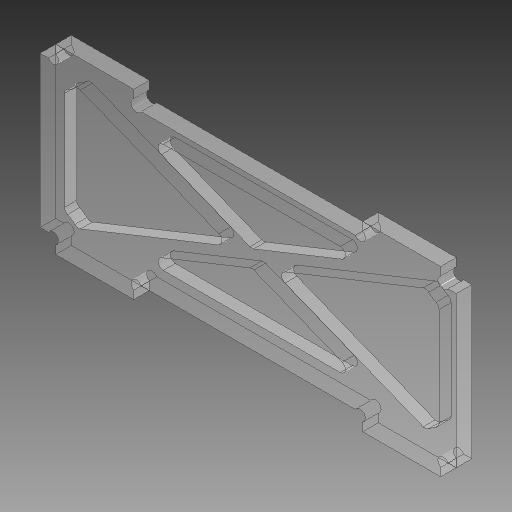
# Autodesk Inventor part: 平行サス板4
Saved by Autodesk Inventor 2020 (Build 240168000, 168)
## iProperties
Created: 2019-09-03
Part Number: 平行サス板4
Material: ポリカーボネート、クリア
Document SubType Name: Modeling
Designer: 雪村
Density: 1.2 g/cm^3
Appearance: ポリカーボネート - クリア
Mass: 5.70734 g
Surface Area: 64.8254 cm^2
Volume: 4.75612 cm^3
Description: ポリカ 3t
Author: 雪村
Autodesk Inventor part; units mm, degrees
ref_plane "YZ Plane" through (0, 0, 0) normal (1, 0, 0) x (0, 1, 0)
ref_plane "XZ Plane" through (0, 0, 0) normal (0, 1, 0) x (-1, 0, 0)
ref_plane "XY Plane" through (0, 0, 0) normal (0, 0, 1) x (1, 0, 0)
sketch "スケッチ1" plane through (0, 0, 0) normal (0, 0, 1) x (1, 0, 0)
  line L0 (0, 0) -> (80, 0)
  line L1 (80, 0) -> (80, 29)
  line L2 (80, 29) -> (0, 29)
  line L3 (0, 29) -> (0, 0)
  line L4 (3, 29) -> (18, 29)
  line L5 (18, 29) -> (18, 32)
  line L6 (18, 32) -> (3, 32)
  line L7 (3, 32) -> (3, 29)
  line L8 (77, 29) -> (62, 29)
  line L9 (62, 29) -> (62, 32)
  line L10 (62, 32) -> (77, 32)
  line L11 (77, 32) -> (77, 29)
  line L12 (3, 0) -> (18, 0)
  line L13 (18, 0) -> (18, -3)
  line L14 (18, -3) -> (3, -3)
  line L15 (3, -3) -> (3, 0)
  line L16 (62, 0) -> (77, 0)
  line L17 (77, 0) -> (77, -3)
  line L18 (77, -3) -> (62, -3)
  line L19 (62, -3) -> (62, 0)
  dimension "d0" = 29
  dimension "d1" = 80
  dimension "d2" = 15
  dimension "d3" = 3
  dimension "d4" = 15
  dimension "d5" = 3
  dimension "d6" = 15
  dimension "d7" = 3
  dimension "d8" = 15
  dimension "d9" = 3
  dimension "d10" = 3
  dimension "d11" = 3
  dimension "d12" = 3
  dimension "d13" = 3
  constraints: 40 end point, 10 horizontal, 10 vertical, 4 point on line
  measures "d0" distance of L1.end L0.end
  measures "d1" distance of L1.end L2.end
  measures "d2" distance of L6.end L5.end
  measures "d3" distance of L5.end L4.end
  measures "d4" distance of L9.end L10.end
  measures "d5" distance of L8.end L9.end
  measures "d6" distance of L13.end L14.end
  measures "d7" distance of L12.end L13.end
  measures "d8" distance of L17.end L18.end
  measures "d9" distance of L16.end L17.end
  measures "d10" distance between parallel lines of L1 L17
  measures "d11" distance between parallel lines of L15 L3
  measures "d12" distance between parallel lines of L3 L7
  measures "d13" distance between parallel lines of L1 L11
extrude "押し出し1" add sketch "スケッチ1" along normal blind 3
sketch "スケッチ2" plane through (0, 0, 3) normal (0, 0, 1) x (1, 0, 0)
  line L0 (3, 29) -> (0, 29) projected
  line L1 (3, 32) -> (3, 29) projected
  line L2 (18, 29) -> (18, 32) projected
  line L3 (62, 29) -> (18, 29) projected
  line L4 (62, 32) -> (62, 29) projected
  line L5 (77, 29) -> (77, 32) projected
  line L6 (80, 29) -> (77, 29) projected
  line L7 (77, 0) -> (80, 0) projected
  line L8 (77, -3) -> (77, 0) projected
  line L9 (62, 0) -> (62, -3) projected
  line L10 (18, 0) -> (62, 0) projected
  line L11 (18, -3) -> (18, 0) projected
  line L12 (0, 0) -> (3, 0) projected
  circle A0 centre (2.5, 29.5) radius 1.05
  circle A1 centre (18.5, 29.5) radius 1.05
  circle A2 centre (61.5, 29.5) radius 1.05
  circle A3 centre (77.5, 29.5) radius 1.05
  circle A4 centre (2.5, -0.5) radius 1.05
  circle A5 centre (18.5, -0.5) radius 1.05
  circle A6 centre (61.5, -0.5) radius 1.05
  circle A7 centre (77.5, -0.5) radius 1.05
  line L13 (3, 0) -> (3, -3) projected
  dimension "d16" = 2.1
  dimension "d17" = 2.1
  dimension "d18" = 2.1
  dimension "d19" = 2.1
  dimension "d20" = 2.1
  dimension "d21" = 2.1
  dimension "d22" = 2.1
  dimension "d23" = 2.1
  dimension "d24" = 0.5
  dimension "d25" = 0.5
  dimension "d26" = 0.5
  dimension "d27" = 0.5
  dimension "d28" = 0.5
  dimension "d29" = 0.5
  dimension "d30" = 0.5
  dimension "d31" = 0.5
  dimension "d32" = 0.5
  dimension "d33" = 0.5
  dimension "d34" = 0.5
  dimension "d35" = 0.5
  dimension "d36" = 0.5
  dimension "d37" = 0.5
  dimension "d38" = 0.5
  dimension "d39" = 0.5
  constraints: 8 centre point
  measures "d16" diameter of A0
  measures "d17" diameter of A1
  measures "d18" diameter of A2
  measures "d19" diameter of A3
  measures "d20" diameter of A4
  measures "d21" diameter of A5
  measures "d22" diameter of A6
  measures "d23" diameter of A7
  measures "d24" distance from line of L0 A0.centre
  measures "d25" distance from line of L1 A0.centre
  measures "d26" distance from line of L3 A1.centre
  measures "d27" distance from line of L2 A1.centre
  measures "d28" distance from line of L3 A2.centre
  measures "d29" distance from line of L4 A2.centre
  measures "d30" distance from line of L6 A3.centre
  measures "d31" distance from line of L5 A3.centre
  measures "d32" distance from line of A4.centre L12
  measures "d33" distance from line of L13 A4.centre
  measures "d34" distance from line of L10 A5.centre
  measures "d35" distance from line of L11 A5.centre
  measures "d36" distance from line of L10 A6.centre
  measures "d37" distance from line of L9 A6.centre
  measures "d38" distance from line of A7.centre L7
  measures "d39" distance from line of L8 A7.centre
extrude "押し出し2" cut sketch "スケッチ2" against normal through all
shell "シェル1" thickness 4 removed faces 2 at (33.1411, 9.6667, 3) at (46.8589, 19.3333, 0)
sketch "スケッチ3" plane through (0, 0, 3) normal (0, 0, 1) x (1, 0, 0)
  line L0 (76, 24.6779) -> (76, 4.3221) projected
  arc A0 (76, 4.3221) -> (72.6779, 1) centre (77.5, -0.5) ccw projected
  line L1 (72.6779, 1) -> (66.3221, 1) projected
  arc A1 (66.3221, 1) -> (59.2082, 4) centre (61.5, -0.5) ccw projected
  line L2 (59.2082, 4) -> (20.7918, 4) projected
  arc A2 (20.7918, 4) -> (13.6779, 1) centre (18.5, -0.5) ccw projected
  line L3 (13.6779, 1) -> (7.3221, 1) projected
  arc A3 (7.3221, 1) -> (4, 4.3221) centre (2.5, -0.5) ccw projected
  line L4 (4, 4.3221) -> (4, 24.6779) projected
  arc A4 (4, 24.6779) -> (7.3221, 28) centre (2.5, 29.5) ccw projected
  line L5 (7.3221, 28) -> (13.6779, 28) projected
  arc A5 (13.6779, 28) -> (20.7918, 25) centre (18.5, 29.5) ccw projected
  line L6 (20.7918, 25) -> (59.2082, 25) projected
  arc A6 (59.2082, 25) -> (66.3221, 28) centre (61.5, 29.5) ccw projected
  line L7 (66.3221, 28) -> (72.6779, 28) projected
  arc A7 (72.6779, 28) -> (76, 24.6779) centre (77.5, 29.5) ccw projected
  arc A8 (77, 30.4233) -> (78.4233, 29) centre (77.5, 29.5) ccw projected
  line L8 (77, 30.4233) -> (77, 32) projected
  line L9 (77, 32) -> (62, 32) projected
  line L10 (62, 32) -> (62, 30.4233) projected
  arc A9 (60.5767, 29) -> (62, 30.4233) centre (61.5, 29.5) ccw projected
  line L11 (60.5767, 29) -> (19.4233, 29) projected
  arc A10 (18, 30.4233) -> (19.4233, 29) centre (18.5, 29.5) ccw projected
  line L12 (18, 30.4233) -> (18, 32) projected
  line L13 (18, 32) -> (3, 32) projected
  line L14 (3, 32) -> (3, 30.4233) projected
  arc A11 (1.5767, 29) -> (3, 30.4233) centre (2.5, 29.5) ccw projected
  line L15 (1.5767, 29) -> (0, 29) projected
  line L16 (0, 29) -> (0, 0) projected
  line L17 (0, 0) -> (1.5767, 0) projected
  arc A12 (3, -1.4233) -> (1.5767, 0) centre (2.5, -0.5) ccw projected
  line L18 (3, -1.4233) -> (3, -3) projected
  line L19 (3, -3) -> (18, -3) projected
  line L20 (18, -3) -> (18, -1.4233) projected
  arc A13 (19.4233, 0) -> (18, -1.4233) centre (18.5, -0.5) ccw projected
  line L21 (19.4233, 0) -> (60.5767, 0) projected
  arc A14 (62, -1.4233) -> (60.5767, 0) centre (61.5, -0.5) ccw projected
  line L22 (62, -1.4233) -> (62, -3) projected
  line L23 (62, -3) -> (77, -3) projected
  line L24 (77, -3) -> (77, -1.4233) projected
  arc A15 (78.4233, 0) -> (77, -1.4233) centre (77.5, -0.5) ccw projected
  line L25 (78.4233, 0) -> (80, 0) projected
  line L26 (80, 0) -> (80, 29) projected
  line L27 (80, 29) -> (78.4233, 29) projected
  line L28 (5.0797, 28.4681) -> (74.9427, 0.5229)
  line L29 (4.5888, 0.3355) -> (74.1647, 28.1659)
  dimension "d43" = 2.2908
  dimension "d44" = 75.2448
  dimension "d45" = 1.496
  dimension "d46" = 74.9356
  constraints: 4 end point, 4 point on line
  measures "d43" distance of L5.start L28.start
  measures "d44" distance of L28.start L28.end
  measures "d45" distance of L7.end L29.end
  measures "d46" distance of L29.start L29.end
rib "リブ1" sketch "スケッチ3" thickness 3 direction (0, 0, -1) depth 3 extend profile no curves L29 L28
sketch "スケッチ4" plane through (0, 0, 3) normal (0, 0, 1) x (1, 0, 0)
  line L0 (73.5799, 2.6836) -> (44.0389, 14.5) projected
  line L1 (44.0389, 14.5) -> (73.5799, 26.3164) projected
  arc A0 (73.5799, 26.3164) -> (76, 24.6779) centre (77.5, 29.5) ccw projected
  line L2 (76, 24.6779) -> (76, 4.3221) projected
  arc A1 (76, 4.3221) -> (73.5799, 2.6836) centre (77.5, -0.5) ccw projected
  line L3 (69.7111, 1) -> (66.3221, 1) projected
  arc A2 (66.3221, 1) -> (65.3799, 2.7325) centre (61.5, -0.5) ccw projected
  line L4 (65.3799, 2.7325) -> (69.7111, 1) projected
  line L5 (14.6201, 26.2675) -> (10.2889, 28) projected
  line L6 (10.2889, 28) -> (13.6779, 28) projected
  arc A3 (13.6779, 28) -> (14.6201, 26.2675) centre (18.5, 29.5) ccw projected
  line L7 (6.4201, 26.3164) -> (35.9611, 14.5) projected
  line L8 (35.9611, 14.5) -> (6.4201, 2.6836) projected
  arc A4 (6.4201, 2.6836) -> (4, 4.3221) centre (2.5, -0.5) ccw projected
  line L9 (4, 4.3221) -> (4, 24.6779) projected
  arc A5 (4, 24.6779) -> (6.4201, 26.3164) centre (2.5, 29.5) ccw projected
  line L10 (69.7111, 28) -> (65.3799, 26.2675) projected
  arc A6 (65.3799, 26.2675) -> (66.3221, 28) centre (61.5, 29.5) ccw projected
  line L11 (66.3221, 28) -> (69.7111, 28) projected
  line L12 (10.2889, 1) -> (14.6201, 2.7325) projected
  arc A7 (14.6201, 2.7325) -> (13.6779, 1) centre (18.5, -0.5) ccw projected
  line L13 (13.6779, 1) -> (10.2889, 1) projected
  arc A8 (60.9197, 4.5166) -> (59.2082, 4) centre (61.5, -0.5) ccw projected
  line L14 (59.2082, 4) -> (20.7918, 4) projected
  arc A9 (20.7918, 4) -> (19.0803, 4.5166) centre (18.5, -0.5) ccw projected
  line L15 (19.0803, 4.5166) -> (40, 12.8845) projected
  line L16 (40, 12.8845) -> (60.9197, 4.5166) projected
  arc A10 (77, 30.4233) -> (78.4233, 29) centre (77.5, 29.5) ccw projected
  line L17 (77, 30.4233) -> (77, 32) projected
  line L18 (77, 32) -> (62, 32) projected
  line L19 (62, 32) -> (62, 30.4233) projected
  arc A11 (60.5767, 29) -> (62, 30.4233) centre (61.5, 29.5) ccw projected
  line L20 (60.5767, 29) -> (19.4233, 29) projected
  arc A12 (18, 30.4233) -> (19.4233, 29) centre (18.5, 29.5) ccw projected
  line L21 (18, 30.4233) -> (18, 32) projected
  line L22 (18, 32) -> (3, 32) projected
  line L23 (3, 32) -> (3, 30.4233) projected
  arc A13 (1.5767, 29) -> (3, 30.4233) centre (2.5, 29.5) ccw projected
  line L24 (1.5767, 29) -> (0, 29) projected
  line L25 (0, 29) -> (0, 0) projected
  line L26 (0, 0) -> (1.5767, 0) projected
  arc A14 (3, -1.4233) -> (1.5767, 0) centre (2.5, -0.5) ccw projected
  line L27 (3, -1.4233) -> (3, -3) projected
  line L28 (3, -3) -> (18, -3) projected
  line L29 (18, -3) -> (18, -1.4233) projected
  arc A15 (19.4233, 0) -> (18, -1.4233) centre (18.5, -0.5) ccw projected
  line L30 (19.4233, 0) -> (60.5767, 0) projected
  arc A16 (62, -1.4233) -> (60.5767, 0) centre (61.5, -0.5) ccw projected
  line L31 (62, -1.4233) -> (62, -3) projected
  line L32 (62, -3) -> (77, -3) projected
  line L33 (77, -3) -> (77, -1.4233) projected
  arc A17 (78.4233, 0) -> (77, -1.4233) centre (77.5, -0.5) ccw projected
  line L34 (78.4233, 0) -> (80, 0) projected
  line L35 (80, 0) -> (80, 29) projected
  line L36 (80, 29) -> (78.4233, 29) projected
  arc A18 (19.0803, 24.4834) -> (20.7918, 25) centre (18.5, 29.5) ccw projected
  line L37 (20.7918, 25) -> (59.2082, 25) projected
  arc A19 (59.2082, 25) -> (60.9197, 24.4834) centre (61.5, 29.5) ccw projected
  line L38 (60.9197, 24.4834) -> (40, 16.1155) projected
  line L39 (40, 16.1155) -> (19.0803, 24.4834) projected
  point P0 (0, 0)
extrude "押し出し3" add sketch "スケッチ4" against normal blind 3 contours L3 A2 L4 | L5 L6 A3 | L10 A6 L11 | L12 A7 L13
fillet "フィレット1" radius 1 20 edges at (20.7918, 4, 1.5) (59.2082, 4, 1.5) (19.0803, 4.5166, 1.5) (40, 12.8845, 1.5) (60.9197, 4.5166, 1.5) (6.4201, 2.6836, 1.5) (4, 4.3221, 1.5) (4, 24.6779, 1.5) (6.4201, 26.3164, 1.5) (35.9611, 14.5, 1.5) (20.7918, 25, 1.5) (19.0803, 24.4834, 1.5) (59.2082, 25, 1.5) (60.9197, 24.4834, 1.5) (40, 16.1155, 1.5) (76, 24.6779, 1.5) (73.5799, 26.3164, 1.5) (76, 4.3221, 1.5) (73.5799, 2.6836, 1.5) (44.0389, 14.5, 1.5)
sketch "スケッチ5" plane through (0, 0, 3) normal (0, 0, 1) x (1, 0, 0)
  line L0 (57.3899, 23.0715) -> (40.3714, 16.2641) projected
  arc A0 (39.6286, 16.2641) -> (40.3714, 16.2641) centre (40, 17.1926) ccw projected
  line L1 (39.6286, 16.2641) -> (22.6101, 23.0715) projected
  arc A1 (22.9815, 25) -> (22.6101, 23.0715) centre (22.9815, 24) ccw projected
  line L2 (22.9815, 25) -> (57.0185, 25) projected
  arc A2 (57.3899, 23.0715) -> (57.0185, 25) centre (57.0185, 24) ccw projected
  line L3 (22.6101, 5.9285) -> (39.6286, 12.7359) projected
  arc A3 (40.3714, 12.7359) -> (39.6286, 12.7359) centre (40, 11.8074) ccw projected
  line L4 (40.3714, 12.7359) -> (57.3899, 5.9285) projected
  arc A4 (57.0185, 4) -> (57.3899, 5.9285) centre (57.0185, 5) ccw projected
  line L5 (57.0185, 4) -> (22.9815, 4) projected
  arc A5 (22.6101, 5.9285) -> (22.9815, 4) centre (22.9815, 5) ccw projected
  line L6 (72.9418, 2.9388) -> (46.3601, 13.5715) projected
  arc A6 (46.3601, 15.4285) -> (46.3601, 13.5715) centre (46.7315, 14.5) ccw projected
  line L7 (46.3601, 15.4285) -> (72.9418, 26.0612) projected
  arc A7 (74.0052, 25.8546) -> (72.9418, 26.0612) centre (73.3132, 25.1327) ccw projected
  arc A8 (74.0052, 25.8546) -> (75.4132, 24.9013) centre (77.5, 29.5) ccw projected
  arc A9 (76, 23.9907) -> (75.4132, 24.9013) centre (75, 23.9907) ccw projected
  line L8 (76, 23.9907) -> (76, 5.0093) projected
  arc A10 (75.4132, 4.0987) -> (76, 5.0093) centre (75, 5.0093) ccw projected
  arc A11 (75.4132, 4.0987) -> (74.0052, 3.1454) centre (77.5, -0.5) ccw projected
  arc A12 (72.9418, 2.9388) -> (74.0052, 3.1454) centre (73.3132, 3.8673) ccw projected
  line L9 (7.0582, 26.0612) -> (33.6399, 15.4285) projected
  arc A13 (33.6399, 13.5715) -> (33.6399, 15.4285) centre (33.2685, 14.5) ccw projected
  line L10 (33.6399, 13.5715) -> (7.0582, 2.9388) projected
  arc A14 (5.9948, 3.1454) -> (7.0582, 2.9388) centre (6.6868, 3.8673) ccw projected
  arc A15 (5.9948, 3.1454) -> (4.5868, 4.0987) centre (2.5, -0.5) ccw projected
  arc A16 (4, 5.0093) -> (4.5868, 4.0987) centre (5, 5.0093) ccw projected
  line L11 (4, 5.0093) -> (4, 23.9907) projected
  arc A17 (4.5868, 24.9013) -> (4, 23.9907) centre (5, 23.9907) ccw projected
  arc A18 (4.5868, 24.9013) -> (5.9948, 25.8546) centre (2.5, 29.5) ccw projected
  arc A19 (7.0582, 26.0612) -> (5.9948, 25.8546) centre (6.6868, 25.1327) ccw projected
  arc A20 (77, 30.4233) -> (78.4233, 29) centre (77.5, 29.5) ccw projected
  line L12 (77, 30.4233) -> (77, 32) projected
  line L13 (77, 32) -> (62, 32) projected
  line L14 (62, 32) -> (62, 30.4233) projected
  arc A21 (60.5767, 29) -> (62, 30.4233) centre (61.5, 29.5) ccw projected
  line L15 (60.5767, 29) -> (19.4233, 29) projected
  arc A22 (18, 30.4233) -> (19.4233, 29) centre (18.5, 29.5) ccw projected
  line L16 (18, 30.4233) -> (18, 32) projected
  line L17 (18, 32) -> (3, 32) projected
  line L18 (3, 32) -> (3, 30.4233) projected
  arc A23 (1.5767, 29) -> (3, 30.4233) centre (2.5, 29.5) ccw projected
  line L19 (1.5767, 29) -> (0, 29) projected
  line L20 (0, 29) -> (0, 0) projected
  line L21 (0, 0) -> (1.5767, 0) projected
  arc A24 (3, -1.4233) -> (1.5767, 0) centre (2.5, -0.5) ccw projected
  line L22 (3, -1.4233) -> (3, -3) projected
  line L23 (3, -3) -> (18, -3) projected
  line L24 (18, -3) -> (18, -1.4233) projected
  arc A25 (19.4233, 0) -> (18, -1.4233) centre (18.5, -0.5) ccw projected
  line L25 (19.4233, 0) -> (60.5767, 0) projected
  arc A26 (62, -1.4233) -> (60.5767, 0) centre (61.5, -0.5) ccw projected
  line L26 (62, -1.4233) -> (62, -3) projected
  line L27 (62, -3) -> (77, -3) projected
  line L28 (77, -3) -> (77, -1.4233) projected
  arc A27 (78.4233, 0) -> (77, -1.4233) centre (77.5, -0.5) ccw projected
  line L29 (78.4233, 0) -> (80, 0) projected
  line L30 (80, 0) -> (80, 29) projected
  line L31 (80, 29) -> (78.4233, 29) projected
  point P0 (0, 0)
extrude "押し出し4" add sketch "スケッチ5" against normal blind 0.7 contours L0 A0 L1 A1 L2 A2 | L3 A3 L4 A4 L5 A5 | L6 A6 L7 A7 A8 A9 L8 A10 A11 A12 | L9 A13 L10 A14 A15 A16 L11 A17 A18 A19
equation "\"d25\" = d24"
equation "\"d26\" = d25"
equation "\"d27\" = d26"
equation "\"d28\" = d26"
equation "\"d29\" = d28"
equation "\"d30\" = d29"
equation "\"d31\" = d30"
equation "\"d32\" = d25"
equation "\"d33\" = d32"
equation "\"d34\" = d33"
equation "\"d35\" = d34"
equation "\"d36\" = d33"
equation "\"d37\" = d36"
equation "\"d38\" = d33"
equation "\"d39\" = d33"
